Tmp v2 (Autodesk Fusion 360 design; units mm, degrees)
Autodesk Fusion 360 part; units mm, degrees
note: some values were not read from the file. Set by a fixed rule: which sketch regions a step uses.
sketch "Sketch1" plane through (0, 0, 0) normal (0, 0, 1) x (1, 0, 0)
  ellipse E0 centre (0, 0) end of major axis (0, 50) minor radius 25
  line L0 (0, -50) -> (0, 50)
  line L1 (25, 0) -> (-25, 0)
  line L2 (-25, 0) -> (25, 0)
  line L3 (0, 0) -> (0, 50)
  dimension "d1" = 100
  dimension "d2" = 50
  constraint coincident E0.centre L3.start
  constraint vertical L0
  constraint coincident E0 L0.start
  constraint coincident E0 L0.end
  constraint coincident E0 L1.start
  constraint coincident E0 L1.end
  measures "d1" distance of E0
  measures "d2" distance of E0
revolve "Revolve1" add sketch "Sketch1" angle 360 about axis through (0, 0, 0) along (0, 1, 0) contours E0 L0 L1 L2 L3 picked at (5.2231, 29.6534)
extrude "Extrude1" add 1 faces at (-1.9321, 0, 6.7067) along direction (0, -1, 0) blind 200
sketch "Sketch2" plane through (0, -200, 0) normal (0, -1, 0) x (1, 0, 0)
  circle A0 centre (0, 0) radius 25
  circle A1 centre (0, 0) radius 20
  line L0 (0, 0) -> (0, 25) construction
  line L1 (0, 0) -> (-5, 24.4949)
  line L2 (0, 0) -> (5, 24.4949)
  line L3 (0, 0) -> (-23.7132, -7.9173)
  line L4 (0, 0) -> (-18.7132, -16.5776)
  line L5 (0, 0) -> (18.7132, -16.5776)
  line L6 (0, 0) -> (23.7132, -7.9173)
  dimension "d6" = 40
  dimension "d9" = 10
  dimension "d10" = 5
  dimension "d12" = 360
  constraint coincident A0.centre A1.centre
  constraint coincident A0 L0.end
  constraint vertical L0
  constraint coincident A0 L1.end
  constraint coincident A0 L2.end
  measures "d6" diameter of A1
  measures "d9" horizontal distance of L1.end L2.end
  measures "d10" horizontal distance of L0.end L1.end
extrude "Extrude2" add sketch "Sketch2" along normal blind 25 contours A0 A1 L1 L2 | A0 A1 L5 L6 | A0 A1 L3 L4
sketch "Sketch3" plane through (0, -225, 0) normal (0, -1, 0) x (1, 0, 0)
  line L0 (4, 19.5959) -> (5, 24.4949)
  arc A0 (5, 24.4949) -> (-5, 24.4949) centre (0, 0) ccw
  line L1 (-5, 24.4949) -> (-4, 19.5959)
  arc A1 (4, 19.5959) -> (-4, 19.5959) centre (0, 0) ccw
  circle A2 centre (0, 0) radius 5
  line L2 (0, 0) -> (-4, 19.5959)
  line L3 (0, 0) -> (4, 19.5959)
  arc A3 (-23.7132, -7.9173) -> (-18.7132, -16.5776) centre (0, 0) ccw
  line L4 (-18.7132, -16.5776) -> (-14.9706, -13.2621)
  arc A4 (-18.9706, -6.3339) -> (-14.9706, -13.2621) centre (0, 0) ccw
  line L5 (-18.9706, -6.3339) -> (-23.7132, -7.9173)
  arc A5 (18.7132, -16.5776) -> (23.7132, -7.9173) centre (0, 0) ccw
  line L6 (23.7132, -7.9173) -> (18.9706, -6.3339)
  arc A6 (14.9706, -13.2621) -> (18.9706, -6.3339) centre (0, 0) ccw
  line L7 (14.9706, -13.2621) -> (18.7132, -16.5776)
  line L8 (0, 0) -> (-18.9706, -6.3339)
  line L9 (0, 0) -> (-14.9706, -13.2621)
  line L10 (0, 0) -> (14.9706, -13.2621)
  line L11 (0, 0) -> (18.9706, -6.3339)
  circle A7 centre (0, 0) radius 3.75
  dimension "d15" = 10
  dimension "d16" = 7.5
  constraint coincident A0.centre A1.centre
  constraint coincident L1.end A1.end
  constraint coincident L0.start A1.start
  constraint coincident A4.start L5.start
  constraint coincident L4.end A4.end
  constraint coincident A6.start L7.start
  constraint coincident L6.end A6.end
  constraint concentric A5 A7
  measures "d15" diameter of A2
  measures "d16" diameter of A7
extrude "Extrude3" add sketch "Sketch3" against normal blind 2.5 contours A1 A2 L2 L3 | A2 L2 L3 A7 | A2 L3 L11 A7 | A2 L2 L8 A7 | A2 L8 L9 A7 | A2 A4 L8 L9 | A2 A6 L10 L11 | A2 L10 L11 A7 | A2 L9 L10 A7
sketch "Sketch4" plane through (0, -225, 0) normal (0, -1, 0) x (1, 0, 0)
  circle A0 centre (0, 0) radius 3.75
  arc A1 (18.7132, -16.5776) -> (23.7132, -7.9173) centre (0, 0) ccw
  line L0 (23.7132, -7.9173) -> (4.7426, -1.5835)
  arc A2 (4.7426, -1.5835) -> (1, 4.899) centre (0, 0) ccw
  line L1 (1, 4.899) -> (5, 24.4949)
  arc A3 (5, 24.4949) -> (-5, 24.4949) centre (0, 0) ccw
  line L2 (-5, 24.4949) -> (-1, 4.899)
  arc A4 (-1, 4.899) -> (-4.7426, -1.5835) centre (0, 0) ccw
  line L3 (-4.7426, -1.5835) -> (-23.7132, -7.9173)
  arc A5 (-23.7132, -7.9173) -> (-18.7132, -16.5776) centre (0, 0) ccw
  line L4 (-18.7132, -16.5776) -> (-3.7426, -3.3155)
  arc A6 (-3.7426, -3.3155) -> (3.7426, -3.3155) centre (0, 0) ccw
  line L5 (3.7426, -3.3155) -> (18.7132, -16.5776)
  line L6 (-5, 24.4949) -> (0, 57.1727)
  line L7 (0, 57.1727) -> (5, 24.4949)
  constraint coincident A3.end L2.start
  constraint coincident L1.end A3.start
extrude "Extrude4" add sketch "Sketch4" against normal up to surface (25 mm away) contours A3 L6 L7
fillet "Fillet1" radius 2.5 2 edges at (-2.5, -200, 40.8338) (2.5, -200, 40.8338)
chamfer "Chamfer1" distance 2 angle 45 2 edges at (-2.5, -225, 40.8338) (2.5, -225, 40.8338)
pattern_circular "C-Pattern1" count 3 over 360 about axis through (0, 0, 0) along (0, -1, 0) of "Extrude4", "Chamfer1"
sketch "Sketch5" plane through (0, -200, 0) normal (0, -1, 0) x (1, 0, 0)
  line L0 (-14.9706, -13.2621) -> (-18.7132, -16.5776)
  arc A0 (-18.7132, -16.5776) -> (18.7132, -16.5776) centre (0, 0) ccw
  line L1 (18.7132, -16.5776) -> (14.9706, -13.2621)
  arc A1 (14.9706, -13.2621) -> (18.9706, -6.3339) centre (0, 0) ccw
  line L2 (18.9706, -6.3339) -> (23.7132, -7.9173)
  arc A2 (23.7132, -7.9173) -> (5, 24.4949) centre (0, 0) ccw
  line L3 (5, 24.4949) -> (4, 19.5959)
  arc A3 (4, 19.5959) -> (-4, 19.5959) centre (0, 0) ccw
  line L4 (-4, 19.5959) -> (-5, 24.4949)
  arc A4 (-5, 24.4949) -> (-23.7132, -7.9173) centre (0, 0) ccw
  line L5 (-23.7132, -7.9173) -> (-18.9706, -6.3339)
  arc A5 (-18.9706, -6.3339) -> (-14.9706, -13.2621) centre (0, 0) ccw
  arc A6 (-18.9706, -6.3339) -> (-14.9706, -13.2621) centre (0, 0) ccw
  circle A7 centre (0, 0) radius 20
  constraint coincident A0.centre A1.centre
  constraint coincident L5.end A7
extrude "Extrude5" add sketch "Sketch5" along normal blind 2.5 contours L0 A0 L1 A7 | L4 A4 L5 A7 | L2 A2 L3 A7
equation "d7 = ( 360 / 3 ) * 1 deg"
equation "d10 = d9 / 2"
